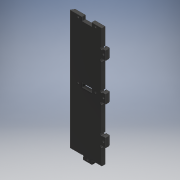
# Autodesk Inventor part: BA03
Saved by Autodesk Inventor 2017 (Build 210142000, 142)
## iProperties
Created: 2019-05-22
Part Number: BA03
Material: Wood (Cherry)
Document SubType Name: Modeling
Designer: Dell
Density: 0.63 g/cm^3
Appearance: Smooth - Black
Mass: 240.222 g
Surface Area: 757.429 cm^2
Volume: 381.304 cm^3
Author: Dell
Autodesk Inventor part; units mm, degrees
ref_plane "YZ Plane" through (0, 0, 0) normal (1, 0, 0) x (0, 1, 0)
ref_plane "XZ Plane" through (0, 0, 0) normal (0, 1, 0) x (-1, 0, 0)
ref_plane "XY Plane" through (0, 0, 0) normal (0, 0, 1) x (1, 0, 0)
sketch "Sketch1" plane through (0, 0, 0) normal (0, 0, 1) x (1, 0, 0)
  line L0 (0, 0) -> (92.075, 0)
  line L1 (92.075, 0) -> (92.075, 9.525)
  line L2 (92.075, 9.525) -> (5.4993, 9.525)
  line L3 (5.4993, 9.525) -> (0, 0)
  dimension "d0" = 92.075
  dimension "d1" = 9.525
  dimension "d2" = 60
  constraints: 8 end point, 2 perpendicular, 1 horizontal
  measures "d0" distance of L0.start L0.end
  measures "d1" distance of L0.end L1.end
  measures "d2" angle of L0 L3
extrude "Extrusion1" add sketch "Sketch1" along normal blind 346.075
sketch "Sketch2" plane through (0, 0, 0) normal (0, -1, 0) x (1, 0, 0)
  line L0 (38.1, 346.075) -> (63.5, 346.075)
  line L1 (63.5, 346.075) -> (63.5, 355.6)
  line L2 (63.5, 355.6) -> (38.1, 355.6)
  line L3 (38.1, 355.6) -> (38.1, 346.075)
  line L4 (0, 346.075) -> (101.6, 346.075)
  line L5 (0, 346.075) -> (92.075, 346.075) projected
  point P0 (0, 0)
  point P1 (50.8, 346.075)
  dimension "d5" = 25.4
  dimension "d6" = 9.525
  dimension "d9" = 101.6
  constraints: 10 end point, 2 midpoint, 2 parallel, 1 collinear, 1 horizontal, 1 perpendicular
  measures "d5" distance of L2.end L1.end
  measures "d6" distance of L1.end L0.end
  measures "d9" distance of L4.start L4.end
extrude "Extrusion2" add sketch "Sketch2" against normal blind 12.7
sketch "Sketch3" plane through (0, 0, 0) normal (0, -1, 0) x (1, 0, 0)
  line L0 (63.5, 346.075) -> (63.5, 355.6) projected
  line L1 (63.5, 355.6) -> (38.1, 355.6) projected
  circle A0 centre (50.8, 350.8375) radius 2.25
  point P0 (0, 0)
  point P1 (50.8, 355.6)
  point P2 (63.5, 350.8375)
  dimension "d10" = 4.5
  constraints: 2 midpoint, 1 centre point, 1 horizontal alignment, 1 vertical alignment
  measures "d10" diameter of A0
extrude "Extrusion3" cut sketch "Sketch3" against normal through all
sketch "Sketch4" plane through (0, 0, 0) normal (0, -1, 0) x (1, 0, 0)
  line L0 (92.075, 0) -> (92.075, 346.075) projected
  line L1 (92.075, 50.8) -> (101.6, 50.8)
  line L2 (101.6, 50.8) -> (101.6, 76.2)
  line L3 (101.6, 76.2) -> (92.075, 76.2)
  line L4 (92.075, 76.2) -> (92.075, 50.8)
  line L5 (92.075, 295.275) -> (101.6, 295.275)
  line L6 (101.6, 295.275) -> (101.6, 269.875)
  line L7 (101.6, 269.875) -> (92.075, 269.875)
  line L8 (92.075, 269.875) -> (92.075, 295.275)
  line L9 (92.075, 185.7375) -> (101.6, 185.7375)
  line L10 (101.6, 185.7375) -> (101.6, 160.3375)
  line L11 (101.6, 160.3375) -> (92.075, 160.3375)
  line L12 (92.075, 160.3375) -> (92.075, 185.7375)
  circle A0 centre (96.8375, 282.575) radius 2.25
  circle A1 centre (96.8375, 173.0375) radius 2.25
  circle A2 centre (96.8375, 63.5) radius 2.25
  point P0 (0, 0)
  point P1 (92.075, 173.0375)
  point P2 (96.8375, 295.275)
  point P3 (96.8375, 185.7375)
  point P4 (96.8375, 76.2)
  point P5 (101.6, 282.575)
  point P6 (101.6, 173.0375)
  point P7 (101.6, 63.5)
  dimension "d13" = 9.525
  dimension "d14" = 25.4
  dimension "d15" = 9.525
  dimension "d16" = 25.4
  dimension "d17" = 9.525
  dimension "d18" = 25.4
  dimension "d19" = 50.8
  dimension "d20" = 50.8
  dimension "d21" = 4.5
  dimension "d22" = 4.5
  dimension "d23" = 4.5
  constraints: 24 end point, 8 midpoint, 6 parallel, 3 centre point, 3 horizontal, 3 horizontal alignment, 3 perpendicular, 3 point on line, 3 vertical alignment
  measures "d13" distance of L3.end L2.end
  measures "d14" distance of L2.end L1.end
  measures "d15" distance of L6.end L7.end
  measures "d16" distance of L5.end L6.end
  measures "d17" distance of L10.end L11.end
  measures "d18" distance of L9.end L10.end
  measures "d19" distance from line of L0.end L5
  measures "d20" distance from line of L0.start L1
  measures "d21" diameter of A0
  measures "d22" diameter of A1
  measures "d23" diameter of A2
extrude "Extrusion4" add sketch "Sketch4" against normal blind 12.7
sketch "Sketch9" plane through (92.075, 0, 295.275) normal (0, 0, 1) x (1, 0, 0)
  line L0 (-92.075, 0) -> (0, 0) projected
  line L1 (-92.075, 0) -> (-92.075, 9.525)
  line L2 (0, 9.525) -> (-86.5757, 9.525) projected
  line L3 (-92.075, 9.525) -> (-86.5757, 9.525)
  line L4 (-86.5757, 9.525) -> (-92.075, 0)
  line L5 (-86.5757, 9.525) -> (-92.075, 0) projected
  constraints: 6 end point, 1 horizontal, 1 vertical
extrude "Extrusion9" [suppressed]
sketch "Sketch10" plane through (92.075, 0, 185.7375) normal (0, 0, 1) x (1, 0, 0)
  line L0 (-81.5677, 12.7) -> (-88.9, 0) projected
  line L1 (-81.5677, 12.7) -> (-88.9, 12.7) projected
  line L2 (-88.9, 12.7) -> (-88.9, 0) projected
  point P0 (-92.075, 0)
extrude "Extrusion10" [suppressed]
sketch "Sketch11" plane through (92.075, 0, 76.2) normal (0, 0, 1) x (1, 0, 0)
  line L0 (-81.5677, 12.7) -> (-88.9, 0) projected
  line L1 (-81.5677, 12.7) -> (-88.9, 12.7) projected
  line L2 (-88.9, 12.7) -> (-88.9, 0) projected
  point P0 (-92.075, 0)
extrude "Extrusion11" [suppressed]
ref_plane "Work Plane1" through (0, 0, 173.0375) normal (0, 0, 1) x (1, 0, 0)
mirror "Mirror1" about plane through (0, 0, 173.0375) normal (0, 0, 1) of "Extrusion1", "Extrusion2", "Extrusion3", "Extrusion4"
sketch "Sketch12" plane through (5.4993, 9.525, 346.075) normal (0, 1, 0) x (1, 0, 0)
  line L0 (58.0007, 0) -> (58.0007, -9.525) projected
  line L1 (58.0007, -9.525) -> (58.0007, 0) projected
  line L2 (58.0007, -9.525) -> (32.6007, -9.525) projected
  line L3 (32.6007, -9.525) -> (58.0007, -9.525) projected
  line L4 (32.6007, 0) -> (32.6007, -9.525) projected
  line L5 (56.1677, 0) -> (30.7677, 0)
  line L6 (86.5757, 0) -> (58.0007, 0) projected
  line L7 (32.6007, -9.525) -> (58.0007, -9.525)
  line L8 (58.0007, -9.525) -> (58.0007, 0)
  line L9 (58.0007, 0) -> (32.6007, 0)
  line L10 (32.6007, 0) -> (32.6007, -9.525)
  point P0 (-5.4993, 346.075)
  constraints: 10 end point, 2 horizontal, 2 parallel, 1 perpendicular, 1 other
extrude "Extrusion12" cut sketch "Sketch12" along normal through all both and the other way through all
sketch "Sketch13" plane through (5.4993, 9.525, 346.075) normal (0, 1, 0) x (1, 0, 0)
  circle A0 centre (18.2879, 6.35) radius 2.25
  line L0 (86.5757, 0) -> (0, 0) projected
  circle A1 centre (68.2879, 6.35) radius 2.25
  line L1 (30.5879, 0) -> (55.9879, 0)
  line L2 (55.9879, 0) -> (55.9879, 9.525)
  line L3 (55.9879, 9.525) -> (30.5879, 9.525)
  line L4 (30.5879, 9.525) -> (30.5879, 0)
  line L5 (18.2879, 6.35) -> (68.2879, 6.35) construction
  point P0 (-5.4993, 346.075)
  point P1 (43.2879, 6.35)
  point P2 (43.2879, 0)
  point P3 (43.2879, 0)
  dimension "d44" = 4.5
  dimension "d45" = 6.35
  dimension "d46" = 4.5
  dimension "d47" = 25.4
  dimension "d48" = 9.525
  dimension "d49" = 50
  constraints: 10 end point, 5 midpoint, 2 centre point, 2 horizontal, 2 parallel, 1 perpendicular, 1 vertical alignment
  measures "d44" diameter of A0
  measures "d45" distance from line of L0 L5.start
  measures "d46" diameter of A1
  measures "d47" distance of L3.end L2.end
  measures "d48" distance of L2.end L1.end
  measures "d49" distance of L5.start L5.end
extrude "Extrusion13" cut sketch "Sketch13" against normal through all
sketch "Sketch14" plane through (92.075, 0, 50.8) normal (0, -1, 0) x (1, 0, 0)
  line L0 (9.525, 109.5375) -> (9.525, 134.9375) projected
  line L1 (-30.5879, 285.75) -> (-55.9879, 285.75) projected
  line L2 (-55.9879, 129.0625) -> (-30.5879, 129.0625)
  line L3 (-30.5879, 129.0625) -> (-30.5879, 119.5375)
  line L4 (-30.5879, 119.5375) -> (-55.9879, 119.5375)
  line L5 (-55.9879, 119.5375) -> (-55.9879, 129.0625)
  point P0 (-92.075, -50.8)
  dimension "d54" = 9.525
  dimension "d55" = 10
  constraints: 8 end point, 2 parallel, 2 vertical alignment, 1 horizontal, 1 perpendicular
  measures "d54" distance of L4.end L2.start
  measures "d55" distance from line of L0.start L4
extrude "Extrusion14" cut sketch "Sketch14" against normal through all
sketch "Sketch15" plane through (92.075, 0, 50.8) normal (0, -1, 0) x (1, 0, 0)
  circle A0 centre (-68.2879, 124.3) radius 2.25
  circle A1 centre (-18.2879, 124.3) radius 2.25
  circle A2 centre (-68.2879, 288.925) radius 2.25 projected
  circle A3 centre (-18.2879, 288.925) radius 2.25 projected
  line L0 (-30.5879, 129.0625) -> (-30.5879, 119.5375) projected
  point P0 (-92.075, -50.8)
  point P1 (-30.5879, 124.3)
  point P2 (-30.5879, 124.3)
  dimension "d56" = 4.5
  dimension "d57" = 4.5
  constraints: 2 centre point, 2 horizontal alignment, 2 midpoint, 2 vertical alignment
  measures "d56" diameter of A0
  measures "d57" diameter of A1
extrude "Extrusion15" cut sketch "Sketch15" against normal through all contours A0 | A1
sketch "Sketch16" plane through (88.9, 9.525, 292.1) normal (0, 1, 0) x (1, 0, 0)
  line L0 (-54.0829, 123.0325) -> (-26.1429, 123.0325)
  line L1 (-26.1429, 123.0325) -> (-26.1429, 110.9675)
  line L2 (-26.1429, 110.9675) -> (-54.0829, 110.9675)
  line L3 (-54.0829, 110.9675) -> (-54.0829, 123.0325)
  line L4 (-88.9, -53.975) -> (-52.8129, -53.975) projected
  line L5 (-54.0829, -53.975) -> (-26.1429, -53.975)
  line L6 (-26.1429, -53.975) -> (-26.1429, -43.18)
  line L7 (-26.1429, -43.18) -> (-54.0829, -43.18)
  line L8 (-54.0829, -43.18) -> (-54.0829, -53.975)
  line L9 (-27.4129, 112.2375) -> (-52.8129, 112.2375) projected
  line L10 (-52.8129, -44.45) -> (-27.4129, -44.45) projected
  line L11 (-52.8129, 112.2375) -> (-52.8129, 121.7625) projected
  circle A0 centre (-53.0451, 294.3451) radius 3.175
  circle A1 centre (-23.1549, 294.3451) radius 3.175
  circle A2 centre (2.2451, 243.5451) radius 3.175
  circle A3 centre (2.2451, 213.6549) radius 3.175
  circle A4 centre (2.2451, 135.5951) radius 3.175
  circle A5 centre (2.2451, 105.7049) radius 3.175
  circle A6 centre (2.2451, 27.6451) radius 3.175
  circle A7 centre (2.2451, -2.2451) radius 3.175
  line L12 (-53.0451, 294.3451) -> (-50.8, 292.1)
  line L13 (-50.8, 301.625) -> (-50.8, 292.1) projected
  line L14 (0, 241.3) -> (2.2451, 243.5451)
  line L15 (12.7, 241.3) -> (3.175, 241.3) projected
  point P0 (-88.9, 292.1)
  point P1 (-40.1129, 112.2375)
  point P2 (-40.1129, 110.9675)
  point P3 (-40.1129, -43.18)
  point P4 (-40.1129, -44.45)
  point P5 (-52.8129, 117)
  point P6 (-54.0829, 117)
  point P7 (0, 0)
  point P8 (0, 25.4)
  point P9 (0, 107.95)
  point P10 (0, 133.35)
  point P11 (0, 215.9)
  point P12 (-25.4, 292.1)
  dimension "d63" = 6.35
  dimension "d64" = 6.35
  dimension "d65" = 6.35
  dimension "d66" = 6.35
  dimension "d67" = 6.35
  dimension "d68" = 6.35
  dimension "d69" = 6.35
  dimension "d70" = 6.35
  dimension "d60" = 1.27
  dimension "d61" = 1.27
  dimension "d62" = 1.27
  dimension "d77" = 45
  dimension "d78" = 45
  constraints: 20 end point, 9 vertical alignment, 6 midpoint, 4 parallel, 3 coincident, 3 point on line, 2 horizontal, 2 horizontal alignment, 2 perpendicular, 24 other
  measures "d60" distance between parallel lines of L2 L9
  measures "d61" distance between parallel lines of L3 L11
  measures "d62" distance between parallel lines of L7 L10
  measures "d77" angle of L13 L12
  measures "d78" angle of L14 L15
extrude "Extrusion16" cut sketch "Sketch16" against normal through all
sketch "Sketch17" plane through (101.6, 9.525, 295.275) normal (0, 1, 0) x (1, 0, 0)
  line L0 (-63.5, 304.8) -> (-38.1, 304.8)
  line L1 (-38.1, 304.8) -> (-38.1, 306.07)
  line L2 (-38.1, 306.07) -> (-63.5, 306.07)
  line L3 (-63.5, 306.07) -> (-63.5, 304.8)
  line L4 (0, 244.475) -> (1.27, 244.475)
  line L5 (1.27, 244.475) -> (1.27, 219.075)
  line L6 (1.27, 219.075) -> (0, 219.075)
  line L7 (0, 219.075) -> (0, 244.475)
  line L8 (0, 134.9375) -> (1.27, 134.9375)
  line L9 (1.27, 134.9375) -> (1.27, 109.5375)
  line L10 (1.27, 109.5375) -> (0, 109.5375)
  line L11 (0, 109.5375) -> (0, 134.9375)
  line L12 (0, 25.4) -> (1.27, 25.4)
  line L13 (1.27, 25.4) -> (1.27, 0)
  line L14 (1.27, 0) -> (0, 0)
  line L15 (0, 0) -> (0, 25.4)
  point P0 (-101.6, 295.275)
  dimension "d73" = 1.27
  dimension "d74" = 1.27
  constraints: 32 end point, 8 parallel, 4 coincident, 4 horizontal, 4 perpendicular, 1 point on line, 1 vertical alignment
  measures "d73" distance between parallel lines of L2 L0
  measures "d74" distance of L4.start L4.end
extrude "Extrusion17" add sketch "Sketch17" against normal up to surface (9.525 mm away) from surface at 0
equation "\"d1\" = Panel_Thickness"
equation "\"d6\" = Panel_Thickness"
equation "\"d13\" = Panel_Thickness"
equation "\"d15\" = Panel_Thickness"
equation "\"d17\" = Panel_Thickness"
equation "\"d48\" = Panel_Thickness"
equation "\"d54\" = Panel_Thickness"
equation "\"d63\" = Tool_Dia"
equation "\"d64\" = d63"
equation "\"d65\" = d63"
equation "\"d66\" = d63"
equation "\"d67\" = d63"
equation "\"d68\" = d63"
equation "\"d69\" = d63"
equation "\"d70\" = d63"
equation "\"d60\" = Fit_Tolerance"
equation "\"d61\" = Fit_Tolerance"
equation "\"d62\" = Fit_Tolerance"
equation "\"d73\" = Fit_Tolerance"
equation "\"d74\" = d73"
equation "\"Panel_Thickness\" = 9.525"
equation "\"Fit_Tolerance\" = 1.27"
equation "\"Tool_Dia\" = 6.35"
body "Solid1"
